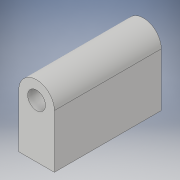
# Autodesk Inventor part: rope guide hole
Saved by Autodesk Inventor 2019 (Build 230136000, 136)
## iProperties
Created: 2018-09-12
Part Number: rope guide hole
Material: Generic
Document SubType Name: Modeling
Designer: HIVE
Density: 1 g/cm^3
Appearance: Default
Author: HIVE
## iProperties of the stored document rope guide hole_3DPrint.ipt
Created: 2018-09-12
Part Number: rope guide hole_3DPrint
Material: Generic
Document SubType Name: Modeling
Designer: HIVE
Density: 1 g/cm^3
Appearance: Default
Author: HIVE
Autodesk Inventor part; units mm, degrees
ref_plane "YZ Plane" through (0, 0, 0) normal (1, 0, 0) x (0, 1, 0)
ref_plane "XZ Plane" through (0, 0, 0) normal (0, 1, 0) x (-1, 0, 0)
ref_plane "XY Plane" through (0, 0, 0) normal (0, 0, 1) x (1, 0, 0)
sketch "Sketch1" plane through (0, 0, 0) normal (0, 0, 1) x (1, 0, 0)
  circle A0 centre (0, 0) radius 2.5
  circle A1 centre (0, 0) radius 5
  line L0 (-4.9556, -0.665) -> (-4.9556, -15)
  line L1 (-4.9556, -15) -> (5, -15)
  line L2 (5, -15) -> (5, 0)
  dimension "d0" = 5
  dimension "d1" = 10
  dimension "d2" = 15
  constraints: 6 end point, 2 centre point, 2 coincident, 2 point on circle, 2 vertical, 1 perpendicular, 1 tangent
  measures "d0" diameter of A0
  measures "d1" diameter of A1
  measures "d2" distance of L1.end L2.end
extrude "Extrusion1" add sketch "Sketch1" along normal blind 30
body "Solid1"
